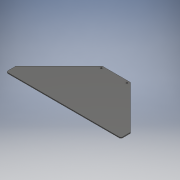
# Autodesk Inventor part: -ZPanel_PCBExtender
Saved by Autodesk Inventor 2018 (Build 220112000, 112)
## iProperties
Created: 2018-11-03
Part Number: -ZPanel_PCBExtender
Material: Epoxy Resin
Document SubType Name: Modeling
Designer: Bradley
Density: 1.14 g/cm^3
Appearance: Smooth - Dark Gray
Author: Bradley
Autodesk Inventor part; units mm, degrees
ref_plane "YZ Plane" through (0, 0, 0) normal (1, 0, 0) x (0, 1, 0)
ref_plane "XZ Plane" through (0, 0, 0) normal (0, 1, 0) x (-1, 0, 0)
ref_plane "XY Plane" through (0, 0, 0) normal (0, 0, 1) x (1, 0, 0)
sketch "Sketch1" plane through (0, 0, 0) normal (0, 0, 1) x (1, 0, 0)
  line L0 (-38, -3.2322) -> (38, -3.2322)
  line L1 (38, -3.2322) -> (38, 3.2322)
  line L2 (38, 3.2322) -> (9.4645, 31.7678)
  line L3 (9.4645, 31.7678) -> (-9.4645, 31.7678)
  line L4 (-9.4645, 31.7678) -> (-38, 3.2322)
  line L5 (-38, 3.2322) -> (-38, -3.2322)
  line L6 (-48, -3.2322) -> (48, -3.2322) construction
  line L7 (48, -3.2322) -> (0, 44.7678) construction
  line L8 (0, 44.7678) -> (-48, -3.2322) construction
  point P0 (0, 0)
  point P1 (0, -3.2322)
  point P2 (0, 31.7678)
  point P3 (38, 0)
  dimension "d0" = 76
  dimension "d1" = 96
  dimension "d2" = 2.5
  dimension "d3" = 35
  constraints: 18 end point, 5 perpendicular, 3 midpoint, 3 vertical alignment, 2 horizontal, 2 parallel, 1 collinear, 1 horizontal alignment
  measures "d0" distance of L0.start L0.end
  measures "d1" distance of L6.start L6.end
  measures "d2" distance between parallel lines of L7 L2
  measures "d3" distance between parallel lines of L0 L3
extrude "Extrusion1" add sketch "Sketch1" along normal mid plane 0.6
sketch "Sketch4" plane through (0, 0, 0.3) normal (0, 0, 1) x (1, 0, 0)
  line L0 (-38, -3.2322) -> (38, -3.2322) projected
  line L1 (38, -3.2322) -> (38, 3.2322) projected
  line L2 (38, 3.2322) -> (9.4645, 31.7678) projected
  line L3 (9.4645, 31.7678) -> (-9.4645, 31.7678) projected
  line L4 (-9.4645, 31.7678) -> (-38, 3.2322) projected
  line L5 (-38, 3.2322) -> (-38, -3.2322) projected
  line L6 (-8.5, 30.2678) -> (8.5, 30.2678) construction
  point P0 (0, 0)
  point P1 (0, 30.2678)
  dimension "d19" = 17
  dimension "d20" = 33.5
  constraints: 2 coincident, 2 end point, 1 horizontal, 1 midpoint, 1 vertical alignment
  measures "d19" distance of L6.start L6.end
  measures "d20" distance between parallel lines of L0 L6
hole "Hole1" at (-8.5, 30.2678, 0.3) at (8.5, 30.2678, 0.3) direction (0, 0, -1) diameter 1 end through all
fillet "Fillet1" radius 1 6 edges at (38, -3.2322, 0) (38, 3.2322, 0) (9.4645, 31.7678, 0) (-9.4645, 31.7678, 0) (-38, 3.2322, 0) (-38, -3.2322, 0)
body "Solid1"
